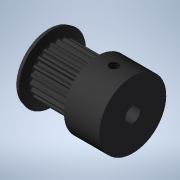
# Autodesk Inventor part: HTPA22S2M100-K-P4_a
Saved by Autodesk Inventor 2021 (Build 250183000, 183)
## iProperties
Created: 2025-03-04
Part Number: HTPA22S2M100-K-P4_a
Material: Generic
Catalog Web Link: www.cadenas.de
Description: HTPA_ _S2M040, HTPA_ _S2M060, HTPA_ _S2M100, HTPB_ _S2M040, HTPB_ _S2M060, HTPB_ _S2M100, HTPK_ _S2M040, HTPK_ _S2M060, HTPK_ _S2M100, HTPN_ _S2M040, HTPN_ _S2M060, HTPN_ _S2M100, HTPT_ _S2M040, HTPT_ _S2M060, HTPM_ _S2M040, HTPM_ _S2M060, HTPP_ _S2M040, HTPP_ _S2M060, HTPS_ _S2M040, HTPS_ _S2M060, HTPS_ _S2M100_a-High Torque Timing Pulleys S2M Type
Vendor: MISUMI
Document SubType Name: Modeling
Designer: psAdmin
Manufacturer: MISUMI
Mass: 3.9017 g
Surface Area: 23.9339 cm^2
Volume: 3.9017 cm^3
Density: 1 g/cm^3
Appearance: PSOLRGB-175-175-175
Category: PARTsolutions
Company: MISUMI
Title: HTPA22S2M100-K-P4
Author: Cadenas PARTsolutions
Comments: High Torque Timing Pulleys S2M Type
PSOL_IDENT_0: {$CADENAS_DATA/23d-libs/misumi/metric/51_timing_pulleys/htpm_s2m/htpa_s2m.prj},734 {VTYP=3D},{NB=HTP
PSOL_IDENT_1: A22S2M100-K-P4_a},{LINA=HTPA22S2M100-K-P4},{NN=HTPA_ _S2M040, HTPA_ _S2M060, HTPA_ _S2M100, HTPB_ _S
PSOL_IDENT_2: 2M040, HTPB_ _S2M060, HTPB_ _S2M100, HTPK_ _S2M040, HTPK_ _S2M060, HTPK_ _S2M100, HTPN_ _S2M040, HTP
PSOL_IDENT_3: N_ _S2M060, HTPN_ _S2M100, HTPT_ _S2M040, HTPT_ _S2M060, HTPM_ _S2M040, HTPM_ _S2M060, HTPP_ _S2M040
PSOL_IDENT_4: , HTPP_ _S2M060, HTPS_ _S2M040, HTPS_ _S2M060, HTPS_ _S2M100_a},{DATE=29.05.2023 09:16:33},{GEOMDATE=
PSOL_IDENT_5: 11.01.2023 01:57:31},{VERSION=},{LINEID=70},{WBVAR=MATP,ST,TNW,PS,SBS,DD,Z,J,Q,R,S,T,ALT1,ALT2,M,QSC
PSOL_IDENT_6: ,QFC,QTC,ALT3,K,KSC,KFC,KTC,ALT4,ZM,ZSC,ZFC,ZTC,ALT5,ALT6,ALT7,FC,ALT8,SRG,ALT9,BTC,TL,ALT10,TPC,ALT
PSOL_IDENT_7: 11,BC,ALT12,SLH,ALT13,BN},{WBNUMERIC=DD,Z,J,Q,R,S,T,QSC,QFC,QTC,K,KSC,KFC,KTC,ZSC,ZFC,ZTC,FC,SRG,BTC
PSOL_IDENT_8: ,TL,BC,SLH,BN}  {NB=HTPA22S2M100-K-P4_a},{LINA=HTPA22S2M100-K-P4},{KT=DUMMY},{PN=HTPA22S2M100-K-P4},
PSOL_IDENT_9: {TYPE=HTPA},{MATP=A2017},{MATPALG= 'A2017','Aluminum Alloy 2000 series','S45CE','1045 Carbon Steel E
PSOL_IDENT_10: quivalent','SUS304','304 Stainless Steel' },{ST=CA},{STALG= 'CA' , 'Clear Anodize', 'BA','Black Anod
PSOL_IDENT_11: ize','HAT','Hard Clear Anodize' , 'ENP' , 'Electroless Nickel Plating' },{NT=22},{TNW=S2M100},{TNWAL
PSOL_IDENT_12: G= 'S2M040', 'S2M060','S2M100' },{BW=10},{PS=K},{PSALG='A','K'},{SBS=P},{SBSALG='H','Round Hole','P'
PSOL_IDENT_13: ,'Round Hole + Tap'},{SHSA= 'H', 'Round Hole','V','Stepped Hole','Y','Both Ends Stepped Hole','WB','
PSOL_IDENT_14: Double Stepped Hole' },{SHSB='H','Round Hole','P','Round Hole + Tap','N','New JIS Keywayed Bore + Ta
PSOL_IDENT_15: p (Standard)','NK','New JIS Keywayed Bore + Tap (width 4.0mm, height 1.8mm)','C','Old JIS Keywayed B
PSOL_IDENT_16: ore + Tap','V','Stepped Hole','F','Stepped Hole (Counterbore holes on the boss side)' },{SHSK='H','R
PSOL_IDENT_17: ound Hole','P','Round Hole + Tap'},{SBSPN=-P4},{DD=4.00},{DDALG=[3:4/1],4.5,[5:6/1]},{DDHA=[3:4/1],4
PSOL_IDENT_18: .5,[5:6/1],6.35,[7:7/1]},{DDHBK=[3:4/1],4.5,[5:6/1]},{DDPA=0},{DDPBK=[3:4/1],4.5,[5:6/1]},{DDNA=0},{
PSOL_IDENT_19: DDNBK=0},{DDNK=0},{DDCA=0},{DDCBK=0},{DDVA=0},{DDVF=[3:4/1]},{DDY=[3:5/1]},{DDWB=[3:3/1]},{Z=0},{ZAL
PSOL_IDENT_20: G=[0]},{ZQRMIN=6},{ZAMAX=0},{ZBMAX=6},{DDZ=4},{J=0.0},{JALG=[0]},{JMAX=0},{JMIN=2},{JPN=},{QRMAX=7},
PSOL_IDENT_21: {QRMIN=6},{WBRMAX=-2.00},{WBQMIN=8},{Q=0},{QALG=[0]},{QPN=},{R=0},{RALG=[0]},{S=0.0},{SALG=[0]},{SPN=
PSOL_IDENT_22: },{SMAX=9},{T=0.0},{TALG=[0]},{TPN=},{TMAX=12},{A=11},{W=15},{L=23},{PD=14.01},{OD=13.50},{D=18},{DA
PSOL_IDENT_23: LG=18},{DE=18},{F=18},{E=11},{BBK=0.000},{TTK=0.0},{TT=1},{WL=23.000},{ALT1=},{ALT1ALG= '','w/o KC90
PSOL_IDENT_24: (Set Screw Angle)','KC90','with KC90 (Set Screw Angle)' },{ANG=120.000},{ALT1PN=},{ALT2=},{ALT2ALG=
PSOL_IDENT_25: '','Not applicable' },{M=N/A},{MALG= 'N/A' },{MFTALG= 'N/A' },{MSALG= 'N/A' },{M3D=0.000},{KDML=0},
PSOL_IDENT_26: {ML=0},{MUL=0},{PITCH=0},{QSC=0.0},{QSCALG=0},{QFC=0.0},{QFCALG=0},{QTC=0.0},{QTCALG=0},{QPCDMIN=0},
PSOL_IDENT_27: {QPCDMINALG=0},{QPCDMAX=14},{ALT2PN=},{ALT3=},{ALT3ALG= '','Not applicable' },{K=0.0},{KALG=0},{KMIN=
PSOL_IDENT_28: 4},{KFTMAX=0.0},{KSMAX=0.0},{KSC=0.0},{KSCALG=0},{KFC=0.0},{KFCALG=0},{KTC=0.0},{KTCALG=0},{KPCDMIN=
PSOL_IDENT_29: 8},{KPCDMINALG=8},{KPCDMAX=0},{KSCMIN=8.0},{KSCMINALG=8},{ALT3PN=},{ALT4=},{ALT4ALG= '','Not applica
PSOL_IDENT_30: ble' },{ALT4MIN=14.5},{ALT4MAX=0.5},{ZM=N/A},{ZMALG= 'N/A' },{ZMSALG= 'N/A' },{ZMFTALG= 'N/A' },{ZMD
PSOL_IDENT_31: D1=0.0},{ZMDD2=0.0},{ZMHH=0.0},{ZSC=0.0},{ZSCALG=[0]},{ZFC=0.0},{ZFCALG=[0]},{ZTC=0.0},{ZTCALG=[0]},
PSOL_IDENT_32: {ZPCDMIN=0},{ZPCDMINALG=0},{ZPCDMAX=7},{ALT4PN=},{ALT5=},{ALT5ALG= '','Flange Attached','NFC','with
PSOL_IDENT_33: NFC (Flange not Attached)' },{ALT5PN=},{ALT6=},{ALT6ALG= '','Not applicable' },{ALT6PN=},{ALT7=},{AL
PSOL_IDENT_34: T7ALG= '','w/o FC (Flange Cut)','FC','with FC (Flange Cut)' },{FC=0.0},{FCALG=0},{FCMIN=14.5},{FCMAX=
PSOL_IDENT_35: 16.0},{ALT7PN=},{ALT8=},{ALT8ALG= '','Not applicable' },{ALT8ALGALG=14},{ALT8DD2=0},{ALT8MM=0},{ALT8
PSOL_IDENT_36: NN=0},{QC=0},{KC=0},{ZC=0},{SRG=0.0},{SRGALG=[0]},{SRGMAX=0},{DD2=0.0},{MM=0.00},{NN=0.00},{ALT8PN=}
PSOL_IDENT_37: ,{ALT9ALG= '','Not applicable' },{ALT9=},{BTC9=6},{TL9=1},{BTC=0},{BTCALG=[0]},{TL=0.0},{TLALG=[0]},
PSOL_IDENT_38: {TLMIN=1.0},{TLMAX=-15.5},{BTCL=0},{BTCD=0},{BTCDALG=11.000},{ALT9PN=},{WLBCTL=23},{ALT10=},{ALT10AL
PSOL_IDENT_39: G= '','w/o TPC (Tapped Hole Dimension)','TPC','with TPC (Tapped Hole Dimension)' },{TPC=N/A},{TPCALG=
PSOL_IDENT_40: 'N/A' },{TPCM=3},{ALT10PN=},{ALT11=},{ALT11ALG= '','Not applicable' },{BC=0.0},{BCALG=0},{BCMIN=6},
PSOL_IDENT_41: {BCMAX=7.5},{BCPLANE=18},{M1WBC=18},{ALT11PN=},{ALT12=},{ALT12ALG= '','w/o SLH (Set Screw Length)','
PSOL_IDENT_42: SLH','with SLH (Set Screw Length)' },{SLH=0},{SLHALG=[0]},{ALT12PN=},{ALT13=},{ALT13ALG= '', 'Not ap
PSOL_IDENT_43: plicable' },{BN=0.0},{BNALG=0},{BNMIN=8.5},{BNMAX=18},{ALT13PN=},{AC=M3x3},{M1=3},{M1L=3},{TAP=0.000
PSOL_IDENT_44: },{KYY=2},{KTT=7},{PLANE=0},{CD=14.5},{SRGCUT=1}
NB: HTPA22S2M100-K-P4_a
NN: HTPA_ _S2M040, HTPA_ _S2M060, HTPA_ _S2M100, HTPB_ _S2M040, HTPB_ _S2M060, HTPB_ _S2M100, HTPK_ _S2M040, HTPK_ _S2M060, HTPK_ _S2M100, HTPN_ _S2M040, HTPN_ _S2M060, HTPN_ _S2M100, HTPT_ _S2M040, HTPT_ _S2M060, HTPM_ _S2M040, HTPM_ _S2M060, HTPP_ _S2M040, HTPP_ _S2M060, HTPS_ _S2M040, HTPS_ _S2M060, HTPS_ _S2M100_a
NT: 22
NBSYN: $PN._a
LINA: HTPA22S2M100-K-P4
CATALOG: Misumi
PN: HTPA22S2M100-K-P4
MATP: Aluminum Alloy 2000 series
ST: Clear Anodize
TNW: S2M100
BW: 10
PS: K
SBS: Round Hole + Tap
DD: 4
Z: 0
J: 0
Q: 0
R: 0
S: 0
T: 0
A: 11
W: 15
L: 23
PD: 14.01
OD: 13.5
D: 18
F: 18
ALT1: w/o KC90 (Set Screw Angle)
ALT2: Not applicable
M: N/A
QSC: 0
QFC: 0
QTC: 0
ALT3: Not applicable
K: 0
KSC: 0
KFC: 0
KTC: 0
ALT4: Not applicable
ZM: N/A
ZSC: 0
ZFC: 0
ZTC: 0
ALT5: Flange Attached
ALT6: Not applicable
ALT7: w/o FC (Flange Cut)
FC: 0
ALT8: Not applicable
SRG: 0
ALT9: Not applicable
BTC: 0
TL: 0
ALT10: w/o TPC (Tapped Hole Dimension)
TPC: N/A
ALT11: Not applicable
BC: 0
ALT12: w/o SLH (Set Screw Length)
SLH: 0
ALT13: Not applicable
BN: 0
AC: M3x3
SUPPLIER: MISUMI
ARTICLENO: HTPA22S2M100-K-P4_a
BOMINFO: HTPA22S2M100-K-P4
CREATOR: CADENAS GmbH
Autodesk Inventor part; units mm, degrees
ref_plane "YZ Plane" through (0, 0, 0) normal (1, 0, 0) x (0, 1, 0)
ref_plane "XZ Plane" through (0, 0, 0) normal (0, 1, 0) x (-1, 0, 0)
ref_plane "XY Plane" through (0, 0, 0) normal (0, 0, 1) x (1, 0, 0)
sketch "_____3" plane through (0, 0, 0) normal (0, 0, 1) x (1, 0, 0)
  line L0 (23, 0) -> (0, 0)
  line L1 (0, 0) -> (0, 5.5)
  line L2 (0, 5.5) -> (1, 5.5)
  line L3 (1, 5.5) -> (1, 6.618348)
  line L4 (1, 6.618348) -> (0.431188, 8.741181)
  line L5 (0.431188, 8.741181) -> (1.397114, 9)
  line L6 (1.397114, 9) -> (2, 6.75)
  line L7 (2, 6.75) -> (13, 6.75)
  line L8 (13, 6.75) -> (13, 7.25)
  line L9 (13, 7.25) -> (13.5, 9)
  line L10 (13.5, 9) -> (23, 9)
  line L11 (23, 9) -> (23, 0)
  line L12 (23, 0) -> (0, 0)
  constraints: 26 end point
revolve "Revolution1" add sketch "_____3" angle 360 about axis through (23, 0, 0) along (1, 0, 0)
sketch "Sketch2" plane through (23, 0, 0) normal (1, 0, 0) x (0, 0, -1)
  point P0 (0, 0)
hole "Hole1" at (23, 0, 0) direction (-1, 0, 0) diameter 4 depth 23
sketch "_____6" plane through (2, 0, 0) normal (1, 0, 0) x (0, 0, -1)
  circle A0 centre (0, 0) radius 13.5
  arc A1 (-6.75, 0) -> (-6.748413, -0.146363) centre (0, 0) ccw
  arc A2 (-6.748413, -0.146363) -> (-6.590165, -0.329578) centre (-6.558458, -0.142243) ccw
  arc A3 (-5.990625, -0.595734) -> (-6.590165, -0.329578) centre (-6.81128, -1.635998) ccw
  arc A4 (-5.953176, -0.663173) -> (-5.990625, -0.595734) centre (-6.052561, -0.674244) ccw
  arc A5 (-5.953176, -0.663173) -> (-5.898868, -1.040894) centre (0, 0) ccw
  arc A6 (-5.9158, -1.116152) -> (-5.898868, -1.040894) centre (-5.997346, -1.058271) ccw
  arc A7 (-6.41607, -1.540436) -> (-5.9158, -1.116152) centre (-6.996289, -0.34923) ccw
  arc A8 (-6.41607, -1.540436) -> (-6.51629, -1.760814) centre (-6.332868, -1.71125) ccw
  arc A9 (-6.51629, -1.760814) -> (-6.476578, -1.901695) centre (0, 0) ccw
  arc A10 (-6.476578, -1.901695) -> (-6.43382, -2.041681) centre (0, 0) ccw
  arc A11 (-6.43382, -2.041681) -> (-6.230364, -2.172892) centre (-6.25272, -1.984212) ccw
  arc A12 (-5.580125, -2.259357) -> (-6.230364, -2.172892) centre (-6.074461, -3.488688) ccw
  arc A13 (-5.525193, -2.313513) -> (-5.580125, -2.259357) centre (-5.617433, -2.352136) ccw
  arc A14 (-5.525193, -2.313513) -> (-5.366669, -2.660633) centre (0, 0) ccw
  arc A15 (-5.361712, -2.737613) -> (-5.366669, -2.660633) centre (-5.456262, -2.705051) ccw
  arc A16 (-5.722183, -3.285653) -> (-5.361712, -2.737613) centre (-6.614501, -2.306167) ccw
  arc A17 (-5.722183, -3.285653) -> (-5.756256, -3.52534) centre (-5.594228, -3.426108) ccw
  arc A18 (-5.756256, -3.52534) -> (-5.678461, -3.649326) centre (0, 0) ccw
  arc A19 (-5.678461, -3.649326) -> (-5.597997, -3.771595) centre (0, 0) ccw
  arc A20 (-5.597997, -3.771595) -> (-5.365816, -3.840171) centre (-5.440423, -3.665432) ccw
  arc A21 (-4.717556, -3.73994) -> (-5.365816, -3.840171) centre (-4.845526, -5.058745) ccw
  arc A22 (-4.649592, -3.776427) -> (-4.717556, -3.73994) centre (-4.727214, -3.839472) ccw
  arc A23 (-4.649592, -3.776427) -> (-4.399694, -4.064824) centre (0, 0) ccw
  arc A24 (-4.373251, -4.137289) -> (-4.399694, -4.064824) centre (-4.473144, -4.132684) ccw
  arc A25 (-4.564719, -4.764686) -> (-4.373251, -4.137289) centre (-5.696845, -4.076271) ccw
  arc A26 (-4.564719, -4.764686) -> (-4.529884, -5.004263) centre (-4.402376, -4.863402) ccw
  arc A27 (-4.529884, -5.004263) -> (-4.42031, -5.10131) centre (0, 0) ccw
  arc A28 (-4.42031, -5.10131) -> (-4.308657, -5.195957) centre (0, 0) ccw
  arc A29 (-4.308657, -5.195957) -> (-4.066561, -5.196342) centre (-4.187377, -5.049701) ccw
  arc A30 (-3.472799, -4.917535) -> (-4.066561, -5.196342) centre (-3.224035, -6.218973) ccw
  arc A31 (-3.397308, -4.933396) -> (-3.472799, -4.917535) centre (-3.454025, -5.015757) ccw
  arc A32 (-3.397308, -4.933396) -> (-3.076282, -5.139707) centre (0, 0) ccw
  arc A33 (-3.030494, -5.201787) -> (-3.076282, -5.139707) centre (-3.127639, -5.225512) ccw
  arc A34 (-3.037448, -5.857713) -> (-3.030494, -5.201787) centre (-4.317664, -5.51614) ccw
  arc A35 (-3.037448, -5.857713) -> (-2.936528, -6.077771) centre (-2.85387, -5.906693) ccw
  arc A36 (-2.936528, -6.077771) -> (-2.804051, -6.140016) centre (0, 0) ccw
  arc A37 (-2.804051, -6.140016) -> (-2.670256, -6.199374) centre (0, 0) ccw
  arc A38 (-2.670256, -6.199374) -> (-2.437858, -6.131537) centre (-2.595093, -6.024873) ccw
  arc A39 (-1.946697, -5.696741) -> (-2.437858, -6.131537) centre (-1.341352, -6.875376) ccw
  arc A40 (-1.869795, -5.690691) -> (-1.946697, -5.696741) centre (-1.90101, -5.785694) ccw
  arc A41 (-1.869795, -5.690691) -> (-1.503648, -5.798202) centre (0, 0) ccw
  arc A42 (-1.442225, -5.844867) -> (-1.503648, -5.798202) centre (-1.528751, -5.895) ccw
  arc A43 (-1.264102, -6.476183) -> (-1.442225, -5.844867) centre (-2.588692, -6.509124) ccw
  arc A44 (-1.264102, -6.476183) -> (-1.105272, -6.658894) centre (-1.074161, -6.471459) ccw
  arc A45 (-1.105272, -6.658894) -> (-0.960625, -6.681295) centre (0, 0) ccw
  arc A46 (-0.960625, -6.681295) -> (-0.815527, -6.700553) centre (0, 0) ccw
  arc A47 (-0.815527, -6.700553) -> (-0.611655, -6.56999) centre (-0.792571, -6.511945) ccw
  arc A48 (-0.262885, -6.014431) -> (-0.611655, -6.56999) centre (0.65, -6.974778) ccw
  arc A49 (-0.190802, -5.98696) -> (-0.262885, -6.014431) centre (-0.193988, -6.08691) ccw
  arc A50 (-0.190802, -5.98696) -> (0.190802, -5.98696) centre (0, 0) ccw
  arc A51 (0.262885, -6.014431) -> (0.190802, -5.98696) centre (0.193988, -6.08691) ccw
  arc A52 (0.611655, -6.56999) -> (0.262885, -6.014431) centre (-0.65, -6.974778) ccw
  arc A53 (0.611655, -6.56999) -> (0.815527, -6.700553) centre (0.792571, -6.511945) ccw
  arc A54 (0.815527, -6.700553) -> (0.960625, -6.681295) centre (0, 0) ccw
  arc A55 (0.960625, -6.681295) -> (1.105272, -6.658894) centre (0, 0) ccw
  arc A56 (1.105272, -6.658894) -> (1.264102, -6.476183) centre (1.074161, -6.471459) ccw
  arc A57 (1.442225, -5.844867) -> (1.264102, -6.476183) centre (2.588692, -6.509124) ccw
  arc A58 (1.503648, -5.798202) -> (1.442225, -5.844867) centre (1.528751, -5.895) ccw
  arc A59 (1.503648, -5.798202) -> (1.869795, -5.690691) centre (0, 0) ccw
  arc A60 (1.946697, -5.696741) -> (1.869795, -5.690691) centre (1.90101, -5.785694) ccw
  arc A61 (2.437858, -6.131536) -> (1.946697, -5.696741) centre (1.341352, -6.875376) ccw
  arc A62 (2.437858, -6.131536) -> (2.670256, -6.199374) centre (2.595093, -6.024873) ccw
  arc A63 (2.670256, -6.199374) -> (2.804051, -6.140016) centre (0, 0) ccw
  arc A64 (2.804051, -6.140016) -> (2.936528, -6.077771) centre (0, 0) ccw
  arc A65 (2.936528, -6.077771) -> (3.037448, -5.857713) centre (2.85387, -5.906693) ccw
  arc A66 (3.030494, -5.201787) -> (3.037448, -5.857713) centre (4.317664, -5.51614) ccw
  arc A67 (3.076282, -5.139707) -> (3.030494, -5.201787) centre (3.127639, -5.225512) ccw
  arc A68 (3.076282, -5.139707) -> (3.397308, -4.933396) centre (0, 0) ccw
  arc A69 (3.472799, -4.917535) -> (3.397308, -4.933396) centre (3.454025, -5.015757) ccw
  arc A70 (4.066561, -5.196342) -> (3.472799, -4.917535) centre (3.224035, -6.218973) ccw
  arc A71 (4.066561, -5.196342) -> (4.308657, -5.195957) centre (4.187377, -5.049701) ccw
  arc A72 (4.308657, -5.195957) -> (4.42031, -5.10131) centre (0, 0) ccw
  arc A73 (4.42031, -5.10131) -> (4.529884, -5.004263) centre (0, 0) ccw
  arc A74 (4.529884, -5.004263) -> (4.564719, -4.764686) centre (4.402376, -4.863402) ccw
  arc A75 (4.373251, -4.137289) -> (4.564719, -4.764686) centre (5.696845, -4.076271) ccw
  arc A76 (4.399694, -4.064824) -> (4.373251, -4.137289) centre (4.473144, -4.132684) ccw
  arc A77 (4.399694, -4.064824) -> (4.649592, -3.776427) centre (0, 0) ccw
  arc A78 (4.717556, -3.73994) -> (4.649592, -3.776427) centre (4.727214, -3.839472) ccw
  arc A79 (5.365816, -3.840171) -> (4.717556, -3.73994) centre (4.845526, -5.058745) ccw
  arc A80 (5.365816, -3.840171) -> (5.597997, -3.771595) centre (5.440423, -3.665432) ccw
  arc A81 (5.597997, -3.771595) -> (5.678461, -3.649326) centre (0, 0) ccw
  arc A82 (5.678461, -3.649326) -> (5.756256, -3.52534) centre (0, 0) ccw
  arc A83 (5.756256, -3.52534) -> (5.722183, -3.285653) centre (5.594228, -3.426108) ccw
  arc A84 (5.361712, -2.737613) -> (5.722183, -3.285653) centre (6.614501, -2.306167) ccw
  arc A85 (5.366669, -2.660633) -> (5.361712, -2.737613) centre (5.456262, -2.705051) ccw
  arc A86 (5.366669, -2.660633) -> (5.525193, -2.313513) centre (0, 0) ccw
  arc A87 (5.580125, -2.259357) -> (5.525193, -2.313513) centre (5.617433, -2.352136) ccw
  arc A88 (6.230364, -2.172892) -> (5.580125, -2.259357) centre (6.074461, -3.488688) ccw
  arc A89 (6.230364, -2.172892) -> (6.43382, -2.041681) centre (6.25272, -1.984212) ccw
  arc A90 (6.43382, -2.041681) -> (6.476578, -1.901695) centre (0, 0) ccw
  arc A91 (6.476578, -1.901695) -> (6.51629, -1.760814) centre (0, 0) ccw
  arc A92 (6.51629, -1.760814) -> (6.41607, -1.540436) centre (6.332868, -1.71125) ccw
  arc A93 (5.9158, -1.116152) -> (6.41607, -1.540436) centre (6.996289, -0.34923) ccw
  arc A94 (5.898868, -1.040894) -> (5.9158, -1.116152) centre (5.997346, -1.058271) ccw
  arc A95 (5.898868, -1.040894) -> (5.953176, -0.663173) centre (0, 0) ccw
  arc A96 (5.990625, -0.595734) -> (5.953176, -0.663173) centre (6.052561, -0.674244) ccw
  arc A97 (6.590165, -0.329578) -> (5.990625, -0.595734) centre (6.81128, -1.635998) ccw
  arc A98 (6.590165, -0.329578) -> (6.748413, -0.146363) centre (6.558458, -0.142243) ccw
  arc A99 (6.748413, -0.146363) -> (6.75, 0) centre (0, 0) ccw
  arc A100 (6.75, 0) -> (6.748413, 0.146363) centre (0, 0) ccw
  arc A101 (6.748413, 0.146363) -> (6.590165, 0.329578) centre (6.558458, 0.142243) ccw
  arc A102 (5.990625, 0.595734) -> (6.590165, 0.329578) centre (6.81128, 1.635998) ccw
  arc A103 (5.953176, 0.663173) -> (5.990625, 0.595734) centre (6.052561, 0.674244) ccw
  arc A104 (5.953176, 0.663173) -> (5.898868, 1.040894) centre (0, 0) ccw
  arc A105 (5.9158, 1.116152) -> (5.898868, 1.040894) centre (5.997346, 1.058271) ccw
  arc A106 (6.41607, 1.540436) -> (5.9158, 1.116152) centre (6.996289, 0.34923) ccw
  arc A107 (6.41607, 1.540436) -> (6.51629, 1.760814) centre (6.332868, 1.71125) ccw
  arc A108 (6.51629, 1.760814) -> (6.476578, 1.901695) centre (0, 0) ccw
  arc A109 (6.476578, 1.901695) -> (6.43382, 2.041681) centre (0, 0) ccw
  arc A110 (6.43382, 2.041681) -> (6.230364, 2.172892) centre (6.25272, 1.984212) ccw
  arc A111 (5.580125, 2.259357) -> (6.230364, 2.172892) centre (6.074461, 3.488688) ccw
  arc A112 (5.525193, 2.313513) -> (5.580125, 2.259357) centre (5.617433, 2.352136) ccw
  arc A113 (5.525193, 2.313513) -> (5.366669, 2.660633) centre (0, 0) ccw
  arc A114 (5.361712, 2.737613) -> (5.366669, 2.660633) centre (5.456262, 2.705051) ccw
  arc A115 (5.722183, 3.285653) -> (5.361712, 2.737613) centre (6.614501, 2.306167) ccw
  arc A116 (5.722183, 3.285653) -> (5.756256, 3.52534) centre (5.594228, 3.426108) ccw
  arc A117 (5.756256, 3.52534) -> (5.678461, 3.649326) centre (0, 0) ccw
  arc A118 (5.678461, 3.649326) -> (5.597997, 3.771595) centre (0, 0) ccw
  arc A119 (5.597997, 3.771595) -> (5.365816, 3.840171) centre (5.440423, 3.665432) ccw
  arc A120 (4.717556, 3.73994) -> (5.365816, 3.840171) centre (4.845526, 5.058745) ccw
  arc A121 (4.649592, 3.776426) -> (4.717556, 3.73994) centre (4.727214, 3.839472) ccw
  arc A122 (4.649592, 3.776426) -> (4.399694, 4.064824) centre (0, 0) ccw
  arc A123 (4.373251, 4.137289) -> (4.399694, 4.064824) centre (4.473144, 4.132684) ccw
  arc A124 (4.564719, 4.764686) -> (4.373251, 4.137289) centre (5.696845, 4.076271) ccw
  arc A125 (4.564719, 4.764686) -> (4.529884, 5.004263) centre (4.402376, 4.863402) ccw
  arc A126 (4.529884, 5.004263) -> (4.42031, 5.10131) centre (0, 0) ccw
  arc A127 (4.42031, 5.10131) -> (4.308657, 5.195957) centre (0, 0) ccw
  arc A128 (4.308657, 5.195957) -> (4.066561, 5.196342) centre (4.187377, 5.049701) ccw
  arc A129 (3.472799, 4.917535) -> (4.066561, 5.196342) centre (3.224035, 6.218973) ccw
  arc A130 (3.397308, 4.933396) -> (3.472799, 4.917535) centre (3.454025, 5.015757) ccw
  arc A131 (3.397308, 4.933396) -> (3.076282, 5.139707) centre (0, 0) ccw
  arc A132 (3.030494, 5.201787) -> (3.076282, 5.139707) centre (3.127639, 5.225512) ccw
  arc A133 (3.037448, 5.857713) -> (3.030494, 5.201787) centre (4.317664, 5.51614) ccw
  arc A134 (3.037448, 5.857713) -> (2.936528, 6.077771) centre (2.85387, 5.906693) ccw
  arc A135 (2.936528, 6.077771) -> (2.804051, 6.140016) centre (0, 0) ccw
  arc A136 (2.804051, 6.140016) -> (2.670256, 6.199374) centre (0, 0) ccw
  arc A137 (2.670256, 6.199374) -> (2.437858, 6.131537) centre (2.595093, 6.024873) ccw
  arc A138 (1.946697, 5.696741) -> (2.437858, 6.131537) centre (1.341352, 6.875376) ccw
  arc A139 (1.869795, 5.690691) -> (1.946697, 5.696741) centre (1.90101, 5.785694) ccw
  arc A140 (1.869795, 5.690691) -> (1.503648, 5.798202) centre (0, 0) ccw
  arc A141 (1.442225, 5.844867) -> (1.503648, 5.798202) centre (1.528751, 5.895) ccw
  arc A142 (1.264102, 6.476183) -> (1.442225, 5.844867) centre (2.588692, 6.509124) ccw
  arc A143 (1.264102, 6.476183) -> (1.105272, 6.658894) centre (1.074161, 6.471459) ccw
  arc A144 (1.105272, 6.658894) -> (0.960625, 6.681295) centre (0, 0) ccw
  arc A145 (0.960625, 6.681295) -> (0.815526, 6.700553) centre (0, 0) ccw
  arc A146 (0.815526, 6.700553) -> (0.611655, 6.56999) centre (0.792571, 6.511945) ccw
  arc A147 (0.262885, 6.014431) -> (0.611655, 6.56999) centre (-0.65, 6.974778) ccw
  arc A148 (0.190802, 5.98696) -> (0.262885, 6.014431) centre (0.193988, 6.08691) ccw
  arc A149 (0.190802, 5.98696) -> (-0.190802, 5.98696) centre (0, 0) ccw
  arc A150 (-0.262885, 6.014431) -> (-0.190802, 5.98696) centre (-0.193988, 6.08691) ccw
  arc A151 (-0.611654, 6.56999) -> (-0.262885, 6.014431) centre (0.65, 6.974778) ccw
  arc A152 (-0.611654, 6.56999) -> (-0.815527, 6.700553) centre (-0.792571, 6.511945) ccw
  arc A153 (-0.815527, 6.700553) -> (-0.960625, 6.681295) centre (0, 0) ccw
  arc A154 (-0.960625, 6.681295) -> (-1.105272, 6.658894) centre (0, 0) ccw
  arc A155 (-1.105272, 6.658894) -> (-1.264102, 6.476183) centre (-1.074161, 6.471459) ccw
  arc A156 (-1.442225, 5.844867) -> (-1.264102, 6.476183) centre (-2.588692, 6.509124) ccw
  arc A157 (-1.503648, 5.798202) -> (-1.442225, 5.844867) centre (-1.528751, 5.895) ccw
  arc A158 (-1.503648, 5.798202) -> (-1.869795, 5.690691) centre (0, 0) ccw
  arc A159 (-1.946697, 5.696741) -> (-1.869795, 5.690691) centre (-1.90101, 5.785694) ccw
  arc A160 (-2.437858, 6.131536) -> (-1.946697, 5.696741) centre (-1.341352, 6.875376) ccw
  arc A161 (-2.437858, 6.131536) -> (-2.670256, 6.199374) centre (-2.595093, 6.024873) ccw
  arc A162 (-2.670256, 6.199374) -> (-2.804051, 6.140016) centre (0, 0) ccw
  arc A163 (-2.804051, 6.140016) -> (-2.936528, 6.077771) centre (0, 0) ccw
  arc A164 (-2.936528, 6.077771) -> (-3.037448, 5.857713) centre (-2.85387, 5.906693) ccw
  arc A165 (-3.030494, 5.201787) -> (-3.037448, 5.857713) centre (-4.317664, 5.51614) ccw
  arc A166 (-3.076282, 5.139707) -> (-3.030494, 5.201787) centre (-3.127639, 5.225512) ccw
  arc A167 (-3.076282, 5.139707) -> (-3.397308, 4.933396) centre (0, 0) ccw
  arc A168 (-3.472799, 4.917535) -> (-3.397308, 4.933396) centre (-3.454025, 5.015757) ccw
  arc A169 (-4.066561, 5.196342) -> (-3.472799, 4.917535) centre (-3.224035, 6.218973) ccw
  arc A170 (-4.066561, 5.196342) -> (-4.308657, 5.195957) centre (-4.187377, 5.049701) ccw
  arc A171 (-4.308657, 5.195957) -> (-4.42031, 5.10131) centre (0, 0) ccw
  arc A172 (-4.42031, 5.10131) -> (-4.529884, 5.004263) centre (0, 0) ccw
  arc A173 (-4.529884, 5.004263) -> (-4.564719, 4.764686) centre (-4.402376, 4.863402) ccw
  arc A174 (-4.373251, 4.137289) -> (-4.564719, 4.764686) centre (-5.696845, 4.076271) ccw
  arc A175 (-4.399694, 4.064824) -> (-4.373251, 4.137289) centre (-4.473144, 4.132684) ccw
  arc A176 (-4.399694, 4.064824) -> (-4.649592, 3.776427) centre (0, 0) ccw
  arc A177 (-4.717556, 3.73994) -> (-4.649592, 3.776427) centre (-4.727214, 3.839472) ccw
  arc A178 (-5.365816, 3.840171) -> (-4.717556, 3.73994) centre (-4.845526, 5.058745) ccw
  arc A179 (-5.365816, 3.840171) -> (-5.597997, 3.771595) centre (-5.440423, 3.665432) ccw
  arc A180 (-5.597997, 3.771595) -> (-5.678461, 3.649326) centre (0, 0) ccw
  arc A181 (-5.678461, 3.649326) -> (-5.756256, 3.525339) centre (0, 0) ccw
  arc A182 (-5.756256, 3.525339) -> (-5.722183, 3.285653) centre (-5.594228, 3.426108) ccw
  arc A183 (-5.361712, 2.737613) -> (-5.722183, 3.285653) centre (-6.614501, 2.306167) ccw
  arc A184 (-5.366669, 2.660633) -> (-5.361712, 2.737613) centre (-5.456262, 2.705051) ccw
  arc A185 (-5.366669, 2.660633) -> (-5.525193, 2.313513) centre (0, 0) ccw
  arc A186 (-5.580125, 2.259357) -> (-5.525193, 2.313513) centre (-5.617433, 2.352136) ccw
  arc A187 (-6.230364, 2.172892) -> (-5.580125, 2.259357) centre (-6.074461, 3.488688) ccw
  arc A188 (-6.230364, 2.172892) -> (-6.43382, 2.041681) centre (-6.25272, 1.984212) ccw
  arc A189 (-6.43382, 2.041681) -> (-6.476578, 1.901695) centre (0, 0) ccw
  arc A190 (-6.476578, 1.901695) -> (-6.51629, 1.760814) centre (0, 0) ccw
  arc A191 (-6.51629, 1.760814) -> (-6.41607, 1.540436) centre (-6.332868, 1.71125) ccw
  arc A192 (-5.9158, 1.116152) -> (-6.41607, 1.540436) centre (-6.996289, 0.34923) ccw
  arc A193 (-5.898868, 1.040894) -> (-5.9158, 1.116152) centre (-5.997346, 1.058271) ccw
  arc A194 (-5.898868, 1.040894) -> (-5.953176, 0.663173) centre (0, 0) ccw
  arc A195 (-5.990625, 0.595734) -> (-5.953176, 0.663173) centre (-6.052561, 0.674244) ccw
  arc A196 (-6.590165, 0.329578) -> (-5.990625, 0.595734) centre (-6.81128, 1.635998) ccw
  arc A197 (-6.590165, 0.329578) -> (-6.748413, 0.146363) centre (-6.558458, 0.142243) ccw
  arc A198 (-6.748413, 0.146363) -> (-6.75, 0) centre (0, 0) ccw
  constraints: 396 point on circle, 199 centre point
extrude "Extrusion1" cut sketch "_____6" along normal blind 11
sketch "_____20" plane through (18, 0, 0) normal (1, 0, 0) x (0, 0, -1)
  line L0 (0, 0) -> (0, 9)
  line L1 (0, 9) -> (1.2295, 9)
  line L2 (1.2295, 9) -> (1.2295, 0)
  line L3 (1.2295, 0) -> (0, 0)
  line L4 (0, 0) -> (0, 9)
  constraints: 10 end point
revolve "Revolution2" cut sketch "_____20" angle 360 about axis through (18, 0, 0) along (0, -1, 0)
thread "Thread1" size "M3x0.5" class "6H" standard "ISO Metric profile" length 7
sketch "_____21" plane through (18, 0, 0) normal (1, 0, 0) x (0, 0, -1)
  line L0 (0, 0) -> (7.794229, -4.5)
  line L1 (7.794229, -4.5) -> (7.179479, -5.564778)
  line L2 (7.179479, -5.564778) -> (-0.61475, -1.064778)
  line L3 (-0.61475, -1.064778) -> (0, 0)
  line L4 (0, 0) -> (7.794229, -4.5)
  constraints: 10 end point
revolve "Revolution3" cut sketch "_____21" angle 360 about axis through (18, 0, 0) along (0, 0.5, 0.8660254)
thread "Thread2" size "M3x0.5" class "6H" standard "ISO Metric profile" length 7 offset 0.3382
ref_plane "C1_XY" through (7.5, 0, 0) normal (1, 0, 0) x (0, 0, -1)
ref_plane "C1_YZ" through (7.5, 0, 0) normal (0, 0, -1) x (0, 1, 0)
ref_plane "C1_ZX" through (7.5, 0, 0) normal (0, 1, 0) x (1, 0, 0)
ref_plane "to_belt_XY" through (7.5, 0, 0) normal (-1, 0, 0) x (0, 0, -1)
ref_plane "to_belt_YZ" through (7.5, 0, 0) normal (0, 0, -1) x (0, -1, 0)
ref_plane "to_belt_ZX" through (7.5, 0, 0) normal (0, -1, 0) x (-1, 0, 0)
ref_plane "to_s1_XY" through (18, 2, 0) normal (0, 1, 0) x (1, 0, 0)
ref_plane "to_s1_YZ" through (18, 2, 0) normal (1, 0, 0) x (0, 0, -1)
ref_plane "to_s1_ZX" through (18, 2, 0) normal (0, 0, -1) x (0, 1, 0)
ref_plane "to_s2_XY" through (18, -1, -1.732051) normal (0, -0.5, -0.8660254) x (1, 0, 0)
ref_plane "to_s2_YZ" through (18, -1, -1.732051) normal (1, 0, 0) x (0, -0.8660254, 0.5)
ref_plane "to_s2_ZX" through (18, -1, -1.732051) normal (0, -0.8660254, 0.5) x (0, -0.5, -0.8660254)
body "Solid1"
